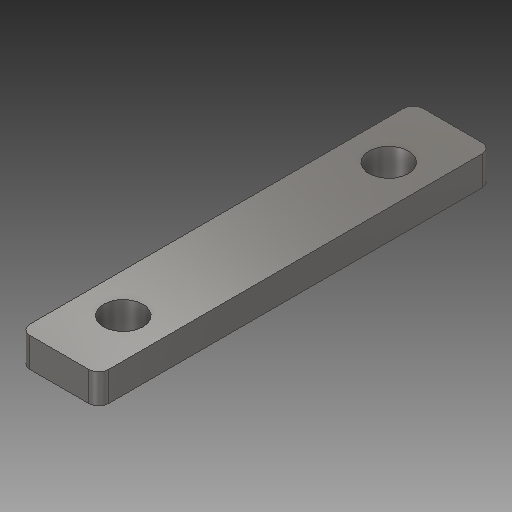
# Autodesk Inventor part: gauge
Saved by Autodesk Inventor 2018 (Build 220112000, 112)
## iProperties
Created: 2018-05-01
Part Number: gauge
Material: Stainless Steel
Document SubType Name: Modeling
Designer: medrimonia
Density: 8 g/cm^3
Appearance: Semi-Polished
Vendor: ???
Mass: 7.05621 g
Surface Area: 9.46265 cm^2
Volume: 0.882027 cm^3
Author: medrimonia
Autodesk Inventor part; units mm, degrees
ref_plane "YZ Plane" through (0, 0, 0) normal (1, 0, 0) x (0, 1, 0)
ref_plane "XZ Plane" through (0, 0, 0) normal (0, 1, 0) x (-1, 0, 0)
ref_plane "XY Plane" through (0, 0, 0) normal (0, 0, 1) x (1, 0, 0)
sketch "Sketch1" plane through (0, 0, 0) normal (0, 1, 0) x (-1, 0, 0)
  line L0 (-4, 20) -> (4, 20)
  line L1 (4, 20) -> (4, -20)
  line L2 (4, -20) -> (-4, -20)
  line L3 (-4, -20) -> (-4, 20)
  line L4 (-4, 20) -> (4, -20) construction
  line L5 (4, 20) -> (-4, -20) construction
  line L6 (0, -20) -> (0, -13.5) construction
  line L7 (0, 20) -> (0, 13.5) construction
  point P0 (0, 0)
  dimension "d0" = 40
  dimension "d1" = 6.5
  dimension "d2" = 8
  constraints: 16 end point, 4 midpoint, 2 coincident, 2 parallel, 2 vertical, 1 collinear, 1 horizontal, 1 perpendicular
  measures "d0" distance of L0.end L1.end
  measures "d1" distance of L6.start L6.end
  measures "d2" distance of L1.end L2.end
extrude "Extrusion1" add sketch "Sketch1" along normal blind 3
hole "Hole1" at (0, 0, -13.5) at (0, 0, 13.5) direction (0, 1, 0) diameter 4 end through all
fillet "Fillet1" radius 1 4 edges at (4, 1.5, 20) (-4, 1.5, 20) (4, 1.5, -20) (-4, 1.5, -20)
equation "\"d0\" = gauge_length"
equation "\"d1\" = hole_2_border"
equation "\"d2\" = gauge_width"
equation "\"d3\" = gauge_thickness"
equation "\"d5\" = hole_diameter"
equation "\"gauge_length\" = 40"
equation "\"gauge_width\" = 8"
equation "\"gauge_thickness\" = 3"
equation "\"hole_diameter\" = 4"
equation "\"hole_2_border\" = 6.5"
body "Solid1"
